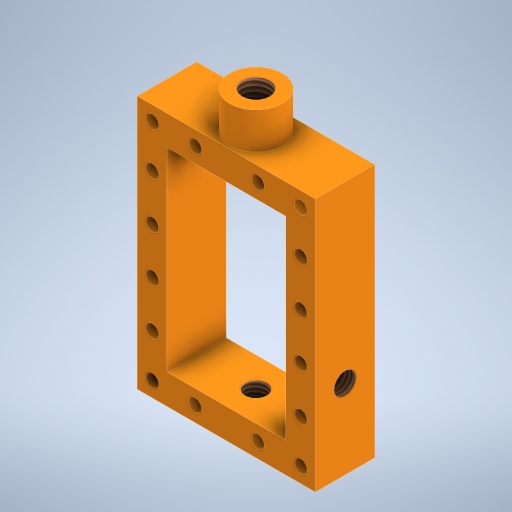
# Autodesk Inventor part: HUDSON-1-32
Saved by Autodesk Inventor 2024.2 (Build 282272000, 272)
## iProperties
Created: 2024-11-02
Part Number: HUDSON-1-32
Material: Generic
Document SubType Name: Modeling
Designer: melim
Density: 1 g/cm^3
Appearance: Orange
Author: melim
Autodesk Inventor part; units mm, degrees
ref_plane "YZ Plane" through (0, 0, 0) normal (1, 0, 0) x (0, 1, 0)
ref_plane "XZ Plane" through (0, 0, 0) normal (0, 1, 0) x (-1, 0, 0)
ref_plane "XY Plane" through (0, 0, 0) normal (0, 0, 1) x (1, 0, 0)
sketch "Sketch1" plane through (0, 0, 0) normal (0, 0, 1) x (1, 0, 0)
  line L0 (27, 38.5) -> (-27, 38.5)
  line L1 (-27, 38.5) -> (-27, -38.5)
  line L2 (-27, -38.5) -> (27, -38.5)
  line L3 (27, -38.5) -> (27, 38.5)
  line L4 (27, 38.5) -> (-27, -38.5) construction
  line L5 (-27, 38.5) -> (27, -38.5) construction
  line L6 (-18, 29.5) -> (18, 29.5)
  line L7 (18, 29.5) -> (18, -29.5)
  line L8 (18, -29.5) -> (-18, -29.5)
  line L9 (-18, -29.5) -> (-18, 29.5)
  line L10 (0, 57.4351) -> (0, -57.4351)
  point P0 (0, 0)
  point P1 (0, 0)
  dimension "d0" = 77
  dimension "d1" = 54
  dimension "d2" = 59
  dimension "d3" = 36
  dimension "d4" = 18
  dimension "d5" = 29.5
  constraints: 22 end point, 4 midpoint, 4 parallel, 2 horizontal, 2 perpendicular, 1 vertical
  measures "d0" distance of L0.end L1.end
  measures "d1" distance of L0.start L0.end
  measures "d2" distance of L6.end L7.end
  measures "d3" distance of L6.start L6.end
  measures "d4" distance from line of L9 point (0, 0)
  measures "d5" distance from line of L6 point (0, 0)
extrude "Extrusion1" add sketch "Sketch1" along normal blind 18 contours L3 L2 L10 L8 L7 L6 L0 | L10 L6 L9 L8 L2 L1 L0
sketch "Sketch2" plane through (0, 0, 18) normal (0, 0, 1) x (1, 0, 0)
  line L0 (27, -38.5) -> (27, 38.5) projected
  line L1 (27, 38.5) -> (-27, 38.5) projected
  line L2 (-27, 38.5) -> (-27, -38.5) projected
  line L3 (-27, -38.5) -> (27, -38.5) projected
  line L4 (18, -29.5) -> (-18, -29.5) projected
  line L5 (-18, -29.5) -> (-18, 29.5) projected
  line L6 (-18, 29.5) -> (18, 29.5) projected
  line L7 (18, 29.5) -> (18, -29.5) projected
  line L8 (-27, 0) -> (26, 0)
  line L9 (0, 38.5) -> (0, -38.5)
  point P0 (0, 0)
  point P1 (-9.5, 34)
  point P2 (9.5, 34)
  point P3 (22.5, 34)
  point P4 (-22.5, 34)
  point P5 (-22.5, 21)
  point P6 (-22.5, 7)
  point P7 (-22.5, -7)
  point P8 (-22.5, -21)
  point P9 (-22.5, -34)
  point P10 (-9.5, -34)
  point P11 (9.5, -34)
  point P12 (22.5, -34)
  point P13 (-0.5, 0)
  point P14 (22.5, 21)
  point P15 (22.5, 7)
  point P16 (22.5, -7)
  point P17 (22.5, -21)
  dimension "d11" = 4.5
  dimension "d14" = 19
  dimension "d15" = 4.5
  dimension "d16" = 13
  dimension "d17" = 4.5
  dimension "d18" = 4.5
  dimension "d19" = 4.5
  dimension "d20" = 13
  dimension "d21" = 4.5
  dimension "d22" = 13
  dimension "d23" = 14
  dimension "d24" = 4.5
  dimension "d25" = 14
  dimension "d26" = 4.5
  dimension "d27" = 4.5
  dimension "d28" = 14
  dimension "d29" = 13
  dimension "d30" = 4.5
  constraints: 7 symmetric about line, 4 end point, 4 midpoint, 1 perpendicular
  measures "d11" distance from line of L1 point (-9.5, 34)
  measures "d14" distance of point (9.5, 34) point (-9.5, 34)
  measures "d15" distance from line of L1 point (9.5, 34)
  measures "d16" distance of point (22.5, 34) point (9.5, 34)
  measures "d17" distance from line of L1 point (22.5, 34)
  measures "d18" distance from line of L1 point (-22.5, 34)
  measures "d19" distance from line of L2 point (-22.5, 34)
  measures "d20" distance of point (-22.5, 34) point (-9.5, 34)
  measures "d21" distance from line of L2 point (-22.5, 21)
  measures "d22" distance of point (-22.5, 21) point (-22.5, 34)
  measures "d23" distance of point (-22.5, 7) point (-22.5, 21)
  measures "d24" distance from line of L2 point (-22.5, 7)
  measures "d25" distance of point (-22.5, -7) point (-22.5, 7)
  measures "d26" horizontal distance of L8.start point (-22.5, -7)
  measures "d27" distance from line of L2 point (-22.5, -21)
  measures "d28" distance of point (-22.5, -7) point (-22.5, -21)
  measures "d29" distance of point (-22.5, -34) point (-22.5, -21)
  measures "d30" distance from line of L2 point (-22.5, -34)
hole "Hole1" at (-9.5, 34, 18) at (9.5, 34, 18) at (22.5, 34, 18) at (-22.5, 34, 18) at (-22.5, 21, 18) at (-22.5, 7, 18) at (-22.5, -7, 18) at (-22.5, -21, 18) at (-22.5, -34, 18) at (-9.5, -34, 18) at (9.5, -34, 18) at (22.5, -34, 18) at (22.5, 21, 18) at (22.5, 7, 18) at (22.5, -7, 18) at (22.5, -21, 18) direction (0, 0, -1) diameter 4 end through all
sketch "Sketch3" plane through (-27, -38.5, 0) normal (0, -1, 0) x (1, 0, 0)
  line L0 (27, 0) -> (27, 18) construction
  line L1 (0, 18) -> (54, 18) projected
  line L2 (0, 0) -> (0, 18) projected
  line L3 (0, 9) -> (54, 9) construction
  line L4 (54, 0) -> (54, 18) projected
  point P0 (27, 9)
  constraints: 4 end point, 4 midpoint
hole "Hole2" at (0, -38.5, 9) direction (0, 1, 0) diameter 6.647 depth 22.2 thread size "M8x1.25" class "6H" standard "ANSI Metric M Profile"
sketch "Sketch4" plane through (-27, 38.5, 0) normal (0, 1, 0) x (1, 0, 0)
  line L0 (27, 0) -> (27, -18) construction
  line L1 (0, -18) -> (54, -18) projected
  line L2 (54, 0) -> (54, -18) projected
  line L3 (54, -9) -> (0, -9) construction
  line L4 (0, 0) -> (0, -18) projected
  circle A0 centre (27, -9) radius 8
  dimension "d45" = 16
  constraints: 4 end point, 4 midpoint, 1 centre point, 1 coincident
  measures "d45" diameter of A0
extrude "Extrusion2" add sketch "Sketch4" along normal blind 11
sketch "Sketch5" plane through (0, 49.5, 9) normal (0, 1, 0) x (1, 0, 0)
  circle A0 centre (0, 0) radius 3.3235 projected
  circle A1 centre (0, 0) radius 8 projected
  point P0 (0, 9)
hole "Hole3" at (0, 49.5, 9) direction (0, -1, 0) diameter 8.376 depth 27.3 thread size "M10x1.5" class "6H" standard "ANSI Metric M Profile"
sketch "Sketch6" plane through (27, -38.5, 0) normal (1, 0, 0) x (0, 0, -1)
  line L0 (0, 0) -> (0, 77) projected
  line L1 (0, 0) -> (0, 77) projected
  line L2 (0, 77) -> (-18, 77) projected
  line L3 (-18, 0) -> (-18, 77) projected
  line L4 (0, 0) -> (-18, 0) projected
  line L5 (0, 29.5) -> (-18, 29.5) projected
  line L6 (0, 19.5) -> (-18, 19.5) projected
  line L7 (0, 9) -> (-18, 9) projected
  line L8 (-9, 0) -> (-9, 77) construction
  point P0 (0, 38.5)
  point P1 (-9, 24)
  constraints: 2 end point, 2 midpoint, 1 point on line
hole "Hole4" at (27, -14.5, 9) direction (-1, 0, 0) diameter 6.647 depth 22.2 thread size "M8x1.25" class "6H" standard "ANSI Metric M Profile"
body "Solid1"
